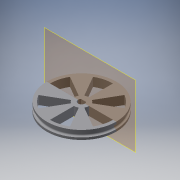
# Autodesk Inventor part: wheel
Saved by Autodesk Inventor 2017 (Build 210142000, 142)
## iProperties
Created: 2018-04-19
Part Number: wheel
Material: Generic
Document SubType Name: Modeling
Designer: winda
Density: 1 g/cm^3
Appearance: Default
Author: winda
Autodesk Inventor part; units mm, degrees
ref_plane "YZ Plane" through (0, 0, 0) normal (1, 0, 0) x (0, 1, 0)
ref_plane "XZ Plane" through (0, 0, 0) normal (0, 1, 0) x (-1, 0, 0)
ref_plane "XY Plane" through (0, 0, 0) normal (0, 0, 1) x (1, 0, 0)
sketch "Sketch1" plane through (0, 0, 0) normal (0, 0, 1) x (1, 0, 0)
  circle A0 centre (0, 0) radius 16
  arc A1 (-1.2247, 0.95) -> (1.2247, 0.95) centre (0, 0) ccw
  line L0 (-1.2247, 0.95) -> (1.2247, 0.95)
  line L1 (-3.5, 0) -> (-14.5, 0)
  line L2 (-3.0311, -1.75) -> (-12.5574, -7.25)
  line L3 (-1.75, -3.0311) -> (-7.25, -12.5574)
  line L4 (0, -3.5) -> (0, -14.5)
  line L5 (1.75, -3.0311) -> (7.25, -12.5574)
  line L6 (3.0311, -1.75) -> (12.5574, -7.25)
  line L7 (3.5, 0) -> (14.5, 0)
  line L8 (3.0311, 1.75) -> (12.5574, 7.25)
  line L9 (1.75, 3.0311) -> (7.25, 12.5574)
  line L10 (0, 3.5) -> (0, 14.5)
  line L11 (-1.75, 3.0311) -> (-7.25, 12.5574)
  line L12 (-3.0311, 1.75) -> (-12.5574, 7.25)
  arc A2 (-3.0311, -1.75) -> (-1.75, -3.0311) centre (0, 0) ccw
  arc A3 (0, -3.5) -> (1.75, -3.0311) centre (0, 0) ccw
  arc A4 (3.0311, -1.75) -> (3.5, 0) centre (0, 0) ccw
  arc A5 (3.0311, 1.75) -> (1.75, 3.0311) centre (0, 0) ccw
  arc A6 (0, 3.5) -> (-1.75, 3.0311) centre (0, 0) ccw
  arc A7 (-3.0311, 1.75) -> (-3.5, 0) centre (0, 0) ccw
  arc A8 (-12.5574, -7.25) -> (-7.25, -12.5574) centre (0, 0) ccw
  arc A9 (0, -14.5) -> (7.25, -12.5574) centre (0, 0) ccw
  arc A10 (12.5574, -7.25) -> (14.5, 0) centre (0, 0) ccw
  arc A11 (12.5574, 7.25) -> (7.25, 12.5574) centre (0, 0) ccw
  arc A12 (0, 14.5) -> (-7.25, 12.5574) centre (0, 0) ccw
  arc A13 (-12.5574, 7.25) -> (-14.5, 0) centre (0, 0) ccw
  dimension "d0" = 32
  dimension "d1" = 3.1
  dimension "d2" = 0.95
  dimension "d18" = 360
  dimension "d20" = 14.5
  constraints: 26 end point, 26 point on circle, 14 centre point, 6 line through centre, 4 coincident, 2 horizontal, 57 other
  measures "d0" diameter of A0
  measures "d1" diameter of A1
  measures "d2" distance from line of point (0, 0) L0
  measures "d20" radius of A13
extrude "Extrusion1" add sketch "Sketch1" along normal blind 4
ref_plane "Work Plane3" through (-1.2247, 0, 0) normal (0, -1, 0) x (1, 0, 0)
sketch "Sketch4" plane through (-1.2247, 0, 0) normal (0, -1, 0) x (1, 0, 0)
  line L0 (17.2247, 4) -> (-14.7753, 4) projected
  line L1 (-14.7753, 0) -> (17.2247, 0) projected
  line L2 (17.2247, 4) -> (-14.7753, 4) construction
  line L3 (1.2247, 4) -> (1.2247, 0) construction
  line L4 (16.2247, 3) -> (17.2247, 3)
  line L5 (17.2247, 3) -> (17.2247, 1)
  line L6 (17.2247, 1) -> (16.2247, 1)
  line L7 (16.2247, 1) -> (16.2247, 3)
  line L8 (17.2247, 0) -> (17.2247, 4) projected
  line L9 (16.2247, 1) -> (16.2247, 0) construction
  line L10 (16.2247, 3) -> (16.2247, 4) construction
  dimension "d10" = 1
  dimension "d11" = 1
  constraints: 14 end point, 3 point on line, 2 collinear, 2 parallel, 2 perpendicular, 1 horizontal, 1 midpoint, 1 vertical
  measures "d10" distance between parallel lines of L1 L6
  measures "d11" distance between parallel lines of L8 L7
revolve "Revolution1" cut sketch "Sketch4" angle 360 about axis through (0, 0, 4) along (0, 0, -1)
fillet "Fillet1" radius 0.6 2 edges at (-15, 0, 3) (-15, 0, 1)
body "Solid1"
